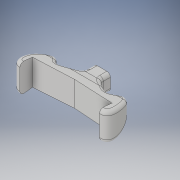
# Autodesk Inventor part: Claw
Saved by Autodesk Inventor 2017 (Build 210142000, 142)
## iProperties
Created: 2018-11-23
Part Number: Claw
Material: Generic
Document SubType Name: Modeling
Designer: Eric the Great
Density: 1 g/cm^3
Appearance: Default
Author: Eric the Great
Autodesk Inventor part; units mm, degrees
ref_plane "YZ Plane" through (0, 0, 0) normal (1, 0, 0) x (0, 1, 0)
ref_plane "XZ Plane" through (0, 0, 0) normal (0, 1, 0) x (-1, 0, 0)
ref_plane "XY Plane" through (0, 0, 0) normal (0, 0, 1) x (1, 0, 0)
sketch "Sketch1" plane through (0, 0, 0) normal (0, 1, 0) x (-1, 0, 0)
  line L0 (28.575, 69.0315) -> (28.575, 60.0315)
  line L1 (28.575, 60.0315) -> (28.575, 69.0315)
  line L2 (28.575, 60.0315) -> (0, 58.3524)
  line L3 (6, 43.7986) -> (6, 38.7324)
  line L4 (0, 0) -> (0, 10.0033)
  line L5 (-28.575, 69.0315) -> (-28.575, 60.0315)
  line L6 (-28.575, 60.0315) -> (-28.575, 69.0315)
  line L7 (-28.575, 60.0315) -> (-28.575, 60.0315)
  line L8 (-28.575, 60.0315) -> (0, 58.3524)
  line L9 (-6, 43.7986) -> (-6, 38.7324)
  line L10 (6, 38.7324) -> (-6, 38.7324)
  spline S0 degree 4 poles (6, 43.7986) (6, 47.0757) (10.9665, 47.9762) (19.208, 58.8303) (23.0741, 41.5275) (33.8195, 52.1578) (36.3846, 69.0315) (28.575, 69.0315) knots 0 0 0 0 0 0.27442 0.455385 0.658982 1 1 1 1 1
  spline S1 degree 4 poles (-6, 43.7986) (-6, 47.0757) (-10.9812, 47.9943) (-23.3932, 64.3487) (-23.0838, 29.9337) (-42.615, 70.9696) (-28.575, 69.0315) knots 0 0 0 0 0 0.27442 0.455385 1 1 1 1 1
  point P0 (18.502, 52.847)
  point P1 (23.2, 48.4338)
  point P2 (30.1758, 51.7081)
  point P3 (11.2515, 49.6471)
  point P4 (-18.502, 52.847)
  point P5 (-23.2, 48.4338)
  point P6 (-30.1758, 51.7081)
  point P7 (-11.2515, 49.6471)
  dimension "d2" = 57.15
  dimension "d3" = 9
  dimension "d7" = 12
  constraints: 22 end point, 9 symmetric about line, 6 vertical, 1 collinear, 1 horizontal, 1 vertical alignment, 12 other
  measures "d2" distance between parallel lines of L0 L5
  measures "d3" distance of L0.start L0.end
  measures "d7" distance of L3.end L9.end
extrude "Extrusion1" add sketch "Sketch1" along normal mid plane 20
sketch "Sketch2" plane through (6, 10, 38.7324) normal (0, 0, -1) x (-1, 0, 0)
  circle A0 centre (6, -10) radius 4.175
  point P0 (6, -10)
  dimension "d4" = 8.35
  constraints: 1 centre point, 1 coincident
  measures "d4" diameter of A0
extrude "Extrusion2" cut sketch "Sketch2" against normal blind 12
sketch "Sketch3" plane through (0, 0, 0) normal (1, 0, 0) x (0, 1, 0)
  line L0 (-10, 43.7986) -> (10, 43.7986) projected
  line L1 (10, 38.7324) -> (10, 43.7986) projected
  line L2 (-10, 38.7324) -> (10, 38.7324) projected
  line L3 (-10, 43.7986) -> (-10, 38.7324) projected
  line L4 (10, 69.0315) -> (-10, 69.0315) projected
  line L5 (-10, 69.0315) -> (10, 69.0315) projected
  arc A0 (6.8594, 51.1774) -> (10, 69.0315) centre (-36.5597, 68.0182) ccw
  line L6 (6, 46.5849) -> (6, 38.7324)
  line L7 (0, 0) -> (0, 3.1446)
  arc A1 (-10, 69.0315) -> (-6.8594, 51.1774) centre (36.5597, 68.0182) ccw
  line L8 (-6, 46.5849) -> (-6, 38.7324)
  arc A2 (6.8594, 51.1774) -> (6, 46.5849) centre (18.7, 46.5849) ccw
  arc A3 (-6, 46.5849) -> (-6.8594, 51.1774) centre (-18.7, 46.5849) ccw
  point P0 (6, 49.1104)
  point P1 (-6, 49.1104)
  dimension "d14" = 12.7
  dimension "d15" = 12.7
  dimension "d16" = 12
  constraints: 10 point on circle, 6 end point, 4 centre point, 4 tangent, 3 point on line, 3 symmetric about line, 1 perpendicular, 1 vertical, 1 other
  measures "d14" radius of A2
  measures "d15" radius of A3
  measures "d16" distance between parallel lines of L8 L6
extrude "Extrusion3" cut sketch "Sketch3" along normal mid plane 400 fills toward (6.05, 42.6586) open curves L6 A2 A0
extrude "Extrusion4" cut sketch "Sketch3" along normal mid plane 400 fills toward (-9.3561, 59.9415) open curves A1 A3 L8
fillet "Fillet2" radius 2.54 24 edges at (25.1856, -6.0601, 47.8189) (17.128, -7.5052, 52.9476) (10.3092, -6.2318, 49.0004) (6.3005, -6, 45.3147) (6, -6, 41.2655) (33.2752, -8.9793, 58.2699) (25.1972, 6.0602, 47.8195) (17.1279, 7.5052, 52.9476) (10.331, 6.2347, 49.0155) (6.3005, 6, 45.3147) (6, 6, 41.2655) (33.2752, 8.9793, 58.2699) (-33.1596, -9.0046, 58.3886) (-17.1096, -7.506, 52.9502) (-10.3081, -6.2316, 48.999) (-6.2982, -6, 45.3103) (-6, -6, 41.2655) (-25.1693, -6.0635, 47.8536) (-17.1097, 7.506, 52.9502) (-10.3081, 6.2316, 48.999) (-6.2982, 6, 45.3103) (-6, 6, 41.2655) (-33.1596, 9.0046, 58.3886) (-25.1815, 6.0636, 47.8542)
body "Solid1"
